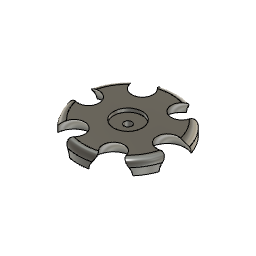
domekit_gheleguen_hub_x6_down_v2 (Autodesk Fusion 360 design; units mm, degrees)
Autodesk Fusion 360 part; units mm, degrees
sketch "Esquisse1" plane through (0, 0, 1) normal (0, 0, 1) x (1, 0, 0)
  circle A0 centre (0, 0) radius 27.75
  dimension "d1" = 55.5
  constraint coincident A0.centre origin
  measures "d1" diameter of A0
extrude "Extrusion1" add sketch "Esquisse1" along normal blind 7.5
ref_plane "Plan de construction3" through (0, 0, 0.5) normal (0, 0, -1) x (-1, 0, 0)
sketch "Esquisse2" plane through (0, 0, 0.5) normal (0, 0, -1) x (1, 0, 0)
  circle A0 centre (22, 0) radius 9.995
  circle A1 centre (0, 0) radius 27.75
  circle A2 centre (0, 0) radius 27.75
  dimension "d4" = 19.99
  dimension "d8" = 22
  measures "d4" diameter of A0
  measures "d8" distance of A1.centre A0.centre
sphere "SpherePrimitive1" cut diameter 19.9 placed x (1, 0, 0) y (0, -1, 0) z (0, 0, -1) at (22, 0, 0.5)
pattern_circular "Réseau C1" count 6 over 360 about axis through (0, 0, 1.75) along (0, 0, 1) of "SpherePrimitive1"
fillet "Congé1" chord length 5 6 edges at (24.0322, -13.875, 8.5) (24.0322, 13.875, 8.5) (0, 27.75, 8.5) (-24.0322, 13.875, 8.5) (-24.0322, -13.875, 8.5) (0, -27.75, 8.5)
hole "Perçage1" at (0, 0, 0.5) direction (0, 0, 1) diameter 4.3 depth 13 tip angle 180
hole "Perçage2" at (0, 0, 8.5) direction (0, 0, -1) diameter 16 depth 2 tip angle 180
